Autodesk Inventor part; units mm, degrees
(part 2 of 2)
sketch "스케치20" plane through (0, 6, 0) normal (0, 1, 0) x (1, 0, 0)
  line L0 (-73.8574, -232.5656) -> (-73.8574, -229.8656) projected
  line L1 (-73.8574, -232.5656) -> (-73.8574, -229.8656) projected
  line L2 (-89.8574, -208.2156) -> (-95.8574, -208.2156) projected
  line L3 (-89.8574, -208.2156) -> (-95.8574, -208.2156) projected
  line L4 (-89.8574, -208.2156) -> (-95.8574, -208.2156) projected
  line L5 (-89.8574, -208.2156) -> (-95.8574, -208.2156) projected
  line L6 (-73.8574, -232.5656) -> (-73.8574, -229.8656) projected
  line L7 (-89.8574, -232.5656) -> (-89.8574, -229.8656) projected
  line L8 (-89.8574, -232.5656) -> (-89.8574, -229.8656) projected
  line L9 (-95.8574, -223.2156) -> (-95.8574, -213.2156) projected
  line L10 (-95.8574, -213.2156) -> (-95.8574, -223.2156) projected
  line L11 (-95.8574, -228.2156) -> (-95.8574, -213.2156) projected
  line L12 (-89.8574, -228.2156) -> (-95.8574, -228.2156) projected
  line L13 (-89.8574, -228.2156) -> (-95.8574, -228.2156) projected
  line L14 (-89.8574, -228.2156) -> (-95.8574, -228.2156) projected
  line L15 (-89.8574, -228.2156) -> (-95.8574, -228.2156) projected
  line L16 (-95.8574, -213.2156) -> (-95.8574, -228.2156) projected
  line L17 (-73.8574, -206.5656) -> (-73.8574, -203.8656) projected
  line L18 (-73.8574, -206.5656) -> (-73.8574, -203.8656) projected
  line L19 (-89.8574, -206.5656) -> (-89.8574, -203.8656) projected
  line L20 (-73.8574, -206.5656) -> (-73.8574, -203.8656) projected
  line L21 (-89.8574, -206.5656) -> (-89.8574, -203.8656) projected
  line L22 (43.6426, -213.2156) -> (43.6426, -223.2156) projected
  line L23 (43.6426, -258.2156) -> (43.6426, -223.2156) projected
  line L24 (43.6426, -203.8656) -> (43.6426, -206.5656) projected
  line L25 (27.6426, -203.8656) -> (27.6426, -206.5656) projected
  line L26 (43.6426, -229.8656) -> (43.6426, -232.5656) projected
  line L27 (27.6426, -229.8656) -> (27.6426, -232.5656) projected
  line L28 (43.6426, -203.8656) -> (43.6426, -206.5656) projected
  line L29 (43.6426, -258.2156) -> (43.6426, -223.2156) projected
  line L30 (43.6426, -213.2156) -> (43.6426, -168.8156) projected
  line L31 (43.6426, -175.4656) -> (43.6426, -178.1656) projected
  line L32 (27.6426, -203.8656) -> (27.6426, -206.5656) projected
  line L33 (27.6426, -229.8656) -> (27.6426, -232.5656) projected
  line L34 (27.6426, -203.8656) -> (27.6426, -206.5656) projected
  line L35 (43.6426, -203.8656) -> (43.6426, -206.5656) projected
  line L36 (27.6426, -229.8656) -> (27.6426, -232.5656) projected
  line L37 (43.6426, -229.8656) -> (43.6426, -232.5656) projected
  line L38 (43.6426, -208.2156) -> (49.6426, -208.2156) projected
  line L39 (43.6426, -208.2156) -> (49.6426, -208.2156) projected
  line L40 (49.6426, -223.2156) -> (49.6426, -213.2156) projected
  line L41 (49.6426, -213.2156) -> (49.6426, -223.2156) projected
  line L42 (43.6426, -228.2156) -> (49.6426, -228.2156) projected
  line L43 (43.6426, -228.2156) -> (49.6426, -228.2156) projected
  line L44 (49.6426, -213.2156) -> (49.6426, -223.2156) projected
  line L45 (43.6426, -228.2156) -> (49.6426, -228.2156) projected
  line L46 (43.6426, -228.2156) -> (49.6426, -228.2156) projected
  line L47 (49.6426, -223.2156) -> (49.6426, -213.2156) projected
  line L48 (43.6426, -208.2156) -> (49.6426, -208.2156) projected
  line L49 (43.6426, -208.2156) -> (49.6426, -208.2156) projected
  line L50 (43.6426, -258.2156) -> (43.6426, -223.2156) projected
  line L51 (43.6426, -258.2156) -> (43.6426, -223.2156) projected
  line L52 (43.6426, -229.8656) -> (43.6426, -232.5656) projected
  line L53 (43.6426, -258.2156) -> (43.6426, -223.2156) projected
  line L54 (43.6426, -258.2156) -> (43.6426, -223.2156) projected
  line L55 (1.8926, -153.8156) -> (1.8926, -173.8156) projected
  line L56 (1.8926, -173.8156) -> (-48.1074, -173.8156) projected
  line L57 (-48.1074, -173.8156) -> (-48.1074, -153.8156) projected
  line L58 (-48.1074, -153.8156) -> (1.8926, -153.8156) projected
  line L59 (-67.2574, -135.1156) -> (-67.2574, -137.3156) projected
  line L60 (-67.2574, -137.3156) -> (-72.4574, -137.3156) projected
  line L61 (-72.4574, -137.3156) -> (-72.4574, -135.1156) projected
  line L62 (-72.4574, -135.1156) -> (-67.2574, -135.1156) projected
  line L63 (21.0426, -135.1156) -> (26.2426, -135.1156) projected
  line L64 (26.2426, -135.1156) -> (26.2426, -137.3156) projected
  line L65 (26.2426, -137.3156) -> (21.0426, -137.3156) projected
  line L66 (21.0426, -137.3156) -> (21.0426, -135.1156) projected
  line L67 (-80.7574, -148.2156) -> (-80.7574, -153.4156) projected
  line L68 (-80.7574, -153.4156) -> (-82.9574, -153.4156) projected
  line L69 (-82.9574, -153.4156) -> (-82.9574, -148.2156) projected
  line L70 (-82.9574, -148.2156) -> (-80.7574, -148.2156) projected
  line L71 (34.5426, -148.2156) -> (36.7426, -148.2156) projected
  line L72 (36.7426, -148.2156) -> (36.7426, -153.4156) projected
  line L73 (36.7426, -153.4156) -> (34.5426, -153.4156) projected
  line L74 (34.5426, -153.4156) -> (34.5426, -148.2156) projected
  line L75 (-8.2304, -181.0703) -> (-8.2304, -248.2156) projected
  line L76 (-8.2304, -248.2156) -> (-38.2304, -248.2156) projected
  line L77 (-38.2304, -248.2156) -> (-38.2304, -181.0703) projected
  arc A0 (-36.6425, -180.6156) -> (-38.2304, -181.0703) centre (-36.6425, -183.6156) ccw projected
  line L78 (-36.6425, -180.6156) -> (-9.8183, -180.6156) projected
  arc A1 (-8.2304, -181.0703) -> (-9.8183, -180.6156) centre (-9.8183, -183.6156) ccw projected
  line L79 (43.6426, -258.2156) -> (43.6426, -223.2156) projected
  line L80 (49.6426, -213.2156) -> (49.6426, -223.2156) projected
  line L81 (43.6426, -213.2156) -> (43.6426, -168.8156) projected
  line L82 (49.6426, -158.8156) -> (49.6426, -168.8156) projected
  line L83 (43.6426, -158.8156) -> (43.6426, -128.2156) projected
  line L84 (43.6426, -128.2156) -> (-3.1074, -128.2156) projected
  line L85 (-3.1074, -128.2156) -> (-3.1074, -122.2156) projected
  line L86 (-43.1074, -122.2156) -> (-3.1074, -122.2156) projected
  line L87 (-43.1074, -128.2156) -> (-43.1074, -122.2156) projected
  line L88 (-43.1074, -128.2156) -> (-89.8574, -128.2156) projected
  line L89 (-89.8574, -128.2156) -> (-89.8574, -158.8156) projected
  line L90 (-95.8574, -223.2156) -> (-95.8574, -213.2156) projected
  line L91 (-89.8574, -223.2156) -> (-89.8574, -258.2156) projected
  line L92 (-89.8574, -258.2156) -> (43.6426, -258.2156) projected
  circle A2 centre (-5.9304, -232.7156) radius 1.35 projected
  circle A3 centre (-5.9304, -210.7156) radius 1.35 projected
  circle A4 centre (-5.9304, -188.7156) radius 1.35 projected
  circle A5 centre (-40.5304, -188.7156) radius 1.35 projected
  circle A6 centre (-40.5304, -232.7156) radius 1.35 projected
  circle A7 centre (-40.5304, -210.7156) radius 1.35 projected
  line L93 (1.8926, -173.8156) -> (1.8926, -153.8156) projected
  line L94 (1.8926, -153.8156) -> (-48.1074, -153.8156) projected
  line L95 (-48.1074, -153.8156) -> (-48.1074, -173.8156) projected
  line L96 (-48.1074, -173.8156) -> (1.8926, -173.8156) projected
  line L97 (-67.2574, -137.3156) -> (-67.2574, -135.1156) projected
  line L98 (-67.2574, -135.1156) -> (-72.4574, -135.1156) projected
  line L99 (-72.4574, -135.1156) -> (-72.4574, -137.3156) projected
  line L100 (-72.4574, -137.3156) -> (-67.2574, -137.3156) projected
  line L101 (26.2426, -135.1156) -> (21.0426, -135.1156) projected
  line L102 (21.0426, -135.1156) -> (21.0426, -137.3156) projected
  line L103 (21.0426, -137.3156) -> (26.2426, -137.3156) projected
  line L104 (26.2426, -137.3156) -> (26.2426, -135.1156) projected
  line L105 (-80.7574, -153.4156) -> (-80.7574, -148.2156) projected
  line L106 (-80.7574, -148.2156) -> (-82.9574, -148.2156) projected
  line L107 (-82.9574, -148.2156) -> (-82.9574, -153.4156) projected
  line L108 (-82.9574, -153.4156) -> (-80.7574, -153.4156) projected
  line L109 (36.7426, -148.2156) -> (34.5426, -148.2156) projected
  line L110 (34.5426, -148.2156) -> (34.5426, -153.4156) projected
  line L111 (34.5426, -153.4156) -> (36.7426, -153.4156) projected
  line L112 (36.7426, -153.4156) -> (36.7426, -148.2156) projected
  line L113 (-8.2304, -181.0703) -> (-8.2304, -248.2156) projected
  arc A8 (-8.2304, -181.0703) -> (-9.8183, -180.6156) centre (-9.8183, -183.6156) ccw projected
  line L114 (-36.6425, -180.6156) -> (-9.8183, -180.6156) projected
  arc A9 (-36.6425, -180.6156) -> (-38.2304, -181.0703) centre (-36.6425, -183.6156) ccw projected
  line L115 (-38.2304, -248.2156) -> (-38.2304, -181.0703) projected
  line L116 (-8.2304, -248.2156) -> (-38.2304, -248.2156) projected
  line L117 (43.6426, -158.8156) -> (43.6426, -128.2156) projected
  line L118 (-89.8574, -258.2156) -> (43.6426, -258.2156) projected
  line L119 (-89.8574, -128.2156) -> (-89.8574, -158.8156) projected
  line L120 (-95.8574, -213.2156) -> (-95.8574, -223.2156) projected
  line L121 (-89.8574, -168.8156) -> (-89.8574, -213.2156) projected
  line L122 (-43.1074, -128.2156) -> (-89.8574, -128.2156) projected
  line L123 (-43.1074, -128.2156) -> (-43.1074, -122.2156) projected
  line L124 (-3.1074, -122.2156) -> (-43.1074, -122.2156) projected
  line L125 (-3.1074, -128.2156) -> (-3.1074, -122.2156) projected
  line L126 (43.6426, -128.2156) -> (-3.1074, -128.2156) projected
  line L127 (43.6426, -258.2156) -> (43.6426, -223.2156) projected
  line L128 (49.6426, -168.8156) -> (49.6426, -158.8156) projected
  line L129 (43.6426, -213.2156) -> (43.6426, -168.8156) projected
  line L130 (49.6426, -223.2156) -> (49.6426, -213.2156) projected
  circle A10 centre (-5.9304, -232.7156) radius 1.35 projected
  circle A11 centre (-5.9304, -210.7156) radius 1.35 projected
  circle A12 centre (-5.9304, -188.7156) radius 1.35 projected
  circle A13 centre (-40.5304, -188.7156) radius 1.35 projected
  circle A14 centre (-40.5304, -232.7156) radius 1.35 projected
  circle A15 centre (-40.5304, -210.7156) radius 1.35 projected
  line L131 (-89.8574, -203.8656) -> (-73.8574, -203.8656) projected
  line L132 (-89.8574, -206.5656) -> (-73.8574, -206.5656) projected
  line L133 (-89.8574, -229.8656) -> (-73.8574, -229.8656) projected
  line L134 (-89.8574, -232.5656) -> (-73.8574, -232.5656) projected
  line L135 (43.6426, -203.8656) -> (27.6426, -203.8656) projected
  line L136 (43.6426, -206.5656) -> (27.6426, -206.5656) projected
  line L137 (43.6426, -229.8656) -> (27.6426, -229.8656) projected
  line L138 (43.6426, -232.5656) -> (27.6426, -232.5656) projected
  line L139 (-82.9574, -207.8156) -> (-80.7574, -207.8156)
  line L140 (-80.7574, -207.8156) -> (-80.7574, -202.6156)
  line L141 (-80.7574, -202.6156) -> (-82.9574, -202.6156)
  line L142 (-82.9574, -202.6156) -> (-82.9574, -207.8156)
  line L143 (-82.9574, -207.8156) -> (-80.7574, -202.6156) construction
  line L144 (-80.7574, -207.8156) -> (-82.9574, -202.6156) construction
  line L145 (-82.9574, -233.9656) -> (-80.7574, -233.9656)
  line L146 (-80.7574, -233.9656) -> (-80.7574, -228.7656)
  line L147 (-80.7574, -228.7656) -> (-82.9574, -228.7656)
  line L148 (-82.9574, -228.7656) -> (-82.9574, -233.9656)
  line L149 (-82.9574, -233.9656) -> (-80.7574, -228.7656) construction
  line L150 (-80.7574, -233.9656) -> (-82.9574, -228.7656) construction
  line L151 (34.5426, -207.8156) -> (36.7426, -207.8156)
  line L152 (36.7426, -207.8156) -> (36.7426, -202.6156)
  line L153 (36.7426, -202.6156) -> (34.5426, -202.6156)
  line L154 (34.5426, -202.6156) -> (34.5426, -207.8156)
  line L155 (34.5426, -207.8156) -> (36.7426, -202.6156) construction
  line L156 (36.7426, -207.8156) -> (34.5426, -202.6156) construction
  line L157 (34.5426, -233.9656) -> (36.7426, -233.9656)
  line L158 (36.7426, -233.9656) -> (36.7426, -228.7656)
  line L159 (36.7426, -228.7656) -> (34.5426, -228.7656)
  line L160 (34.5426, -228.7656) -> (34.5426, -233.9656)
  line L161 (34.5426, -233.9656) -> (36.7426, -228.7656) construction
  line L162 (36.7426, -233.9656) -> (34.5426, -228.7656) construction
  line L163 (43.6426, -213.2156) -> (49.6426, -213.2156) projected
  line L164 (43.6426, -223.2156) -> (49.6426, -223.2156) projected
  line L165 (43.6426, -223.2156) -> (49.6426, -223.2156) projected
  line L166 (43.6426, -213.2156) -> (49.6426, -213.2156) projected
  line L167 (43.6426, -158.8156) -> (43.6426, -128.2156) projected
  line L168 (43.6426, -158.8156) -> (43.6426, -128.2156) projected
  line L169 (43.6426, -213.2156) -> (43.6426, -168.8156) projected
  line L170 (43.6426, -213.2156) -> (43.6426, -168.8156) projected
  line L171 (43.6426, -158.8156) -> (43.6426, -128.2156) projected
  line L172 (43.6426, -158.8156) -> (43.6426, -128.2156) projected
  line L173 (43.6426, -213.2156) -> (43.6426, -168.8156) projected
  line L174 (43.6426, -258.2156) -> (43.6426, -223.2156) projected
  line L175 (43.6426, -158.8156) -> (49.6426, -158.8156) projected
  line L176 (43.6426, -168.8156) -> (49.6426, -168.8156) projected
  line L177 (43.6426, -168.8156) -> (49.6426, -168.8156) projected
  line L178 (43.6426, -158.8156) -> (49.6426, -158.8156) projected
  line L179 (-89.8574, -223.2156) -> (-89.8574, -258.2156) projected
  line L180 (-89.8574, -168.8156) -> (-95.8574, -168.8156) projected
  line L181 (-95.8574, -158.8156) -> (-95.8574, -168.8156) projected
  line L182 (-89.8574, -158.8156) -> (-95.8574, -158.8156) projected
  line L183 (-89.8574, -158.8156) -> (-95.8574, -158.8156) projected
  line L184 (-95.8574, -168.8156) -> (-95.8574, -158.8156) projected
  line L185 (-89.8574, -168.8156) -> (-95.8574, -168.8156) projected
  line L186 (-89.8574, -168.8156) -> (-89.8574, -213.2156) projected
  line L187 (-89.8574, -223.2156) -> (-95.8574, -223.2156) projected
  line L188 (-89.8574, -213.2156) -> (-95.8574, -213.2156) projected
  line L189 (-89.8574, -213.2156) -> (-95.8574, -213.2156) projected
  line L190 (-89.8574, -223.2156) -> (-95.8574, -223.2156) projected
  point P0 (0, 0)
  point P1 (43.6426, -173.8156)
  point P2 (-81.8574, -205.2156)
  point P3 (-81.8574, -231.3656)
  point P4 (35.6426, -205.2156)
  point P5 (35.6426, -231.3656)
  dimension "d155" = 2.2
  dimension "d156" = 5.2
  dimension "d157" = 2.2
  dimension "d158" = 5.2
  dimension "d159" = 2.2
  dimension "d160" = 5.2
  dimension "d161" = 2.2
  dimension "d162" = 5.2
  constraints: 48 end point, 8 midpoint, 8 parallel, 4 horizontal, 4 perpendicular, 7 other
  measures "d155" distance of L141.end L140.end
  measures "d156" distance of L140.end L139.end
  measures "d157" distance of L147.end L146.end
  measures "d158" distance of L146.end L145.end
  measures "d159" distance of L153.end L152.end
  measures "d160" distance of L152.end L151.end
  measures "d161" distance of L159.end L158.end
  measures "d162" distance of L158.end L157.end
extrude "돌출18" cut sketch "스케치20" against normal blind 16 contours L146 L145 L148 L134 | L134 L148 L133 L146 | L133 L148 L147 L146 | L158 L157 L160 L138 | L138 L160 L137 L158 | L137 L160 L159 L158 | L142 L131 L140 L132 | L132 L140 L139 L142 | L142 L141 L140 L131 | L152 L151 L154 L136 | L136 L154 L135 L152 | L135 L154 L153 L152
sketch "스케치22" plane through (0, 6, 0) normal (0, 1, 0) x (1, 0, 0)
  line L0 (36.7426, -207.8156) -> (34.5426, -207.8156) projected
  line L1 (34.5426, -207.8156) -> (34.5426, -202.6156) projected
  line L2 (34.5426, -202.6156) -> (36.7426, -202.6156) projected
  line L3 (36.7426, -202.6156) -> (36.7426, -207.8156) projected
  line L4 (-80.7574, -233.9656) -> (-82.9574, -233.9656) projected
  line L5 (-82.9574, -233.9656) -> (-82.9574, -228.7656) projected
  line L6 (-82.9574, -228.7656) -> (-80.7574, -228.7656) projected
  line L7 (-80.7574, -228.7656) -> (-80.7574, -233.9656) projected
  line L8 (36.7426, -233.9656) -> (34.5426, -233.9656) projected
  line L9 (34.5426, -233.9656) -> (34.5426, -228.7656) projected
  line L10 (34.5426, -228.7656) -> (36.7426, -228.7656) projected
  line L11 (36.7426, -228.7656) -> (36.7426, -233.9656) projected
  line L12 (-80.7574, -207.8156) -> (-82.9574, -207.8156) projected
  line L13 (-82.9574, -207.8156) -> (-82.9574, -202.6156) projected
  line L14 (-82.9574, -202.6156) -> (-80.7574, -202.6156) projected
  line L15 (-80.7574, -202.6156) -> (-80.7574, -207.8156) projected
  line L16 (1.8926, -153.8156) -> (1.8926, -173.8156) projected
  line L17 (1.8926, -173.8156) -> (-48.1074, -173.8156) projected
  line L18 (-48.1074, -173.8156) -> (-48.1074, -153.8156) projected
  line L19 (-48.1074, -153.8156) -> (1.8926, -153.8156) projected
  line L20 (34.5426, -148.2156) -> (36.7426, -148.2156) projected
  line L21 (36.7426, -148.2156) -> (36.7426, -153.4156) projected
  line L22 (36.7426, -153.4156) -> (34.5426, -153.4156) projected
  line L23 (34.5426, -153.4156) -> (34.5426, -148.2156) projected
  line L24 (-80.7574, -148.2156) -> (-80.7574, -153.4156) projected
  line L25 (-80.7574, -153.4156) -> (-82.9574, -153.4156) projected
  line L26 (-82.9574, -153.4156) -> (-82.9574, -148.2156) projected
  line L27 (-82.9574, -148.2156) -> (-80.7574, -148.2156) projected
  line L28 (36.7426, -179.4156) -> (34.5426, -179.4156) projected
  line L29 (34.5426, -179.4156) -> (34.5426, -174.2156) projected
  line L30 (34.5426, -174.2156) -> (36.7426, -174.2156) projected
  line L31 (36.7426, -174.2156) -> (36.7426, -179.4156) projected
  line L32 (21.0426, -135.1156) -> (26.2426, -135.1156) projected
  line L33 (26.2426, -135.1156) -> (26.2426, -137.3156) projected
  line L34 (26.2426, -137.3156) -> (21.0426, -137.3156) projected
  line L35 (21.0426, -137.3156) -> (21.0426, -135.1156) projected
  line L36 (-67.2574, -135.1156) -> (-67.2574, -137.3156) projected
  line L37 (-67.2574, -137.3156) -> (-72.4574, -137.3156) projected
  line L38 (-72.4574, -137.3156) -> (-72.4574, -135.1156) projected
  line L39 (-72.4574, -135.1156) -> (-67.2574, -135.1156) projected
  line L40 (-80.7574, -179.4156) -> (-82.9574, -179.4156) projected
  line L41 (-82.9574, -179.4156) -> (-82.9574, -174.2156) projected
  line L42 (-82.9574, -174.2156) -> (-80.7574, -174.2156) projected
  line L43 (-80.7574, -174.2156) -> (-80.7574, -179.4156) projected
  line L44 (-8.2304, -181.0703) -> (-8.2304, -248.2156) projected
  line L45 (-8.2304, -248.2156) -> (-38.2304, -248.2156) projected
  line L46 (-38.2304, -248.2156) -> (-38.2304, -181.0703) projected
  arc A0 (-36.6425, -180.6156) -> (-38.2304, -181.0703) centre (-36.6425, -183.6156) ccw projected
  line L47 (-36.6425, -180.6156) -> (-9.8183, -180.6156) projected
  arc A1 (-8.2304, -181.0703) -> (-9.8183, -180.6156) centre (-9.8183, -183.6156) ccw projected
  line L48 (43.6426, -258.2156) -> (43.6426, -223.2156) projected
  line L49 (49.6426, -213.2156) -> (49.6426, -223.2156) projected
  line L50 (43.6426, -213.2156) -> (43.6426, -168.8156) projected
  line L51 (49.6426, -158.8156) -> (49.6426, -168.8156) projected
  line L52 (43.6426, -158.8156) -> (43.6426, -128.2156) projected
  line L53 (43.6426, -128.2156) -> (-3.1074, -128.2156) projected
  line L54 (-3.1074, -128.2156) -> (-3.1074, -122.2156) projected
  line L55 (-43.1074, -122.2156) -> (-3.1074, -122.2156) projected
  line L56 (-43.1074, -128.2156) -> (-43.1074, -122.2156) projected
  line L57 (-43.1074, -128.2156) -> (-89.8574, -128.2156) projected
  line L58 (-89.8574, -128.2156) -> (-89.8574, -158.8156) projected
  line L59 (-95.8574, -223.2156) -> (-95.8574, -213.2156) projected
  line L60 (-89.8574, -223.2156) -> (-89.8574, -258.2156) projected
  line L61 (-89.8574, -258.2156) -> (43.6426, -258.2156) projected
  circle A2 centre (-5.9304, -232.7156) radius 1.35 projected
  circle A3 centre (-5.9304, -210.7156) radius 1.35 projected
  circle A4 centre (-5.9304, -188.7156) radius 1.35 projected
  circle A5 centre (-40.5304, -188.7156) radius 1.35 projected
  circle A6 centre (-40.5304, -232.7156) radius 1.35 projected
  circle A7 centre (-40.5304, -210.7156) radius 1.35 projected
  line L62 (1.8926, -188.7156) -> (21.8926, -188.7156)
  line L63 (21.8926, -188.7156) -> (21.8926, -201.7156)
  line L64 (21.8926, -201.7156) -> (1.8926, -201.7156)
  line L65 (1.8926, -201.7156) -> (1.8926, -188.7156)
  line L66 (-48.1074, -188.7156) -> (-68.1074, -188.7156)
  line L67 (-68.1074, -188.7156) -> (-68.1074, -201.7156)
  line L68 (-68.1074, -201.7156) -> (-48.1074, -201.7156)
  line L69 (-48.1074, -201.7156) -> (-48.1074, -188.7156)
  line L70 (21.8926, -188.7156) -> (36.8926, -188.7156)
  line L71 (36.8926, -188.7156) -> (36.8926, -196.7156)
  line L72 (36.8926, -196.7156) -> (21.8926, -196.7156)
  line L73 (21.8926, -196.7156) -> (21.8926, -188.7156)
  line L74 (-68.1074, -188.7156) -> (-83.1074, -188.7156)
  line L75 (-83.1074, -188.7156) -> (-83.1074, -196.7156)
  line L76 (-83.1074, -196.7156) -> (-68.1074, -196.7156)
  line L77 (-68.1074, -196.7156) -> (-68.1074, -188.7156)
  line L78 (43.6426, -223.2156) -> (49.6426, -223.2156) projected
  line L79 (43.6426, -213.2156) -> (49.6426, -213.2156) projected
  line L80 (43.6426, -168.8156) -> (49.6426, -168.8156) projected
  line L81 (43.6426, -158.8156) -> (49.6426, -158.8156) projected
  line L82 (-89.8574, -158.8156) -> (-95.8574, -158.8156) projected
  line L83 (-95.8574, -168.8156) -> (-95.8574, -158.8156) projected
  line L84 (-89.8574, -168.8156) -> (-95.8574, -168.8156) projected
  line L85 (-89.8574, -168.8156) -> (-89.8574, -213.2156) projected
  line L86 (-89.8574, -213.2156) -> (-95.8574, -213.2156) projected
  line L87 (-89.8574, -223.2156) -> (-95.8574, -223.2156) projected
  point P0 (0, 0)
  dimension "d168" = 20
  dimension "d169" = 13
  dimension "d170" = 20
  dimension "d171" = 15
  dimension "d172" = 8
  dimension "d173" = 15
  dimension "d174" = 8
  constraints: 32 end point, 8 parallel, 4 horizontal, 4 perpendicular, 2 point on line
  measures "d168" distance of L63.end L64.end
  measures "d169" distance of L62.end L63.end
  measures "d170" distance of L68.end L67.end
  measures "d171" distance of L71.end L72.end
  measures "d172" distance of L70.end L71.end
  measures "d173" distance of L76.end L75.end
  measures "d174" distance of L75.end L74.end
extrude "돌출19" cut sketch "스케치22" against normal blind 10 contours L70 L71 L72 L63 | L67 L76 L75 L74
sketch "스케치23" plane through (0, 6, 0) normal (0, 1, 0) x (1, 0, 0)
  line L0 (21.8926, -196.7156) -> (21.8926, -188.7156) projected
  line L1 (21.8926, -188.7156) -> (36.8926, -188.7156) projected
  line L2 (36.8926, -188.7156) -> (36.8926, -196.7156) projected
  line L3 (36.8926, -196.7156) -> (21.8926, -196.7156) projected
  line L4 (-68.1074, -188.7156) -> (-68.1074, -196.7156) projected
  line L5 (-68.1074, -196.7156) -> (-83.1074, -196.7156) projected
  line L6 (-83.1074, -196.7156) -> (-83.1074, -188.7156) projected
  line L7 (-83.1074, -188.7156) -> (-68.1074, -188.7156) projected
  line L8 (36.7426, -207.8156) -> (34.5426, -207.8156) projected
  line L9 (34.5426, -207.8156) -> (34.5426, -202.6156) projected
  line L10 (34.5426, -202.6156) -> (36.7426, -202.6156) projected
  line L11 (36.7426, -202.6156) -> (36.7426, -207.8156) projected
  line L12 (-80.7574, -233.9656) -> (-82.9574, -233.9656) projected
  line L13 (-82.9574, -233.9656) -> (-82.9574, -228.7656) projected
  line L14 (-82.9574, -228.7656) -> (-80.7574, -228.7656) projected
  line L15 (-80.7574, -228.7656) -> (-80.7574, -233.9656) projected
  line L16 (36.7426, -233.9656) -> (34.5426, -233.9656) projected
  line L17 (34.5426, -233.9656) -> (34.5426, -228.7656) projected
  line L18 (34.5426, -228.7656) -> (36.7426, -228.7656) projected
  line L19 (36.7426, -228.7656) -> (36.7426, -233.9656) projected
  line L20 (-80.7574, -207.8156) -> (-82.9574, -207.8156) projected
  line L21 (-82.9574, -207.8156) -> (-82.9574, -202.6156) projected
  line L22 (-82.9574, -202.6156) -> (-80.7574, -202.6156) projected
  line L23 (-80.7574, -202.6156) -> (-80.7574, -207.8156) projected
  line L24 (1.8926, -153.8156) -> (1.8926, -173.8156) projected
  line L25 (1.8926, -173.8156) -> (-48.1074, -173.8156) projected
  line L26 (-48.1074, -173.8156) -> (-48.1074, -153.8156) projected
  line L27 (-48.1074, -153.8156) -> (1.8926, -153.8156) projected
  line L28 (34.5426, -148.2156) -> (36.7426, -148.2156) projected
  line L29 (36.7426, -148.2156) -> (36.7426, -153.4156) projected
  line L30 (36.7426, -153.4156) -> (34.5426, -153.4156) projected
  line L31 (34.5426, -153.4156) -> (34.5426, -148.2156) projected
  line L32 (-80.7574, -148.2156) -> (-80.7574, -153.4156) projected
  line L33 (-80.7574, -153.4156) -> (-82.9574, -153.4156) projected
  line L34 (-82.9574, -153.4156) -> (-82.9574, -148.2156) projected
  line L35 (-82.9574, -148.2156) -> (-80.7574, -148.2156) projected
  line L36 (36.7426, -179.4156) -> (34.5426, -179.4156) projected
  line L37 (34.5426, -179.4156) -> (34.5426, -174.2156) projected
  line L38 (34.5426, -174.2156) -> (36.7426, -174.2156) projected
  line L39 (36.7426, -174.2156) -> (36.7426, -179.4156) projected
  line L40 (21.0426, -135.1156) -> (26.2426, -135.1156) projected
  line L41 (26.2426, -135.1156) -> (26.2426, -137.3156) projected
  line L42 (26.2426, -137.3156) -> (21.0426, -137.3156) projected
  line L43 (21.0426, -137.3156) -> (21.0426, -135.1156) projected
  line L44 (-67.2574, -135.1156) -> (-67.2574, -137.3156) projected
  line L45 (-67.2574, -137.3156) -> (-72.4574, -137.3156) projected
  line L46 (-72.4574, -137.3156) -> (-72.4574, -135.1156) projected
  line L47 (-72.4574, -135.1156) -> (-67.2574, -135.1156) projected
  line L48 (-80.7574, -179.4156) -> (-82.9574, -179.4156) projected
  line L49 (-82.9574, -179.4156) -> (-82.9574, -174.2156) projected
  line L50 (-82.9574, -174.2156) -> (-80.7574, -174.2156) projected
  line L51 (-80.7574, -174.2156) -> (-80.7574, -179.4156) projected
  line L52 (-8.2304, -181.0703) -> (-8.2304, -248.2156) projected
  line L53 (-8.2304, -248.2156) -> (-38.2304, -248.2156) projected
  line L54 (-38.2304, -248.2156) -> (-38.2304, -181.0703) projected
  arc A0 (-36.6425, -180.6156) -> (-38.2304, -181.0703) centre (-36.6425, -183.6156) ccw projected
  line L55 (-36.6425, -180.6156) -> (-9.8183, -180.6156) projected
  arc A1 (-8.2304, -181.0703) -> (-9.8183, -180.6156) centre (-9.8183, -183.6156) ccw projected
  line L56 (43.6426, -258.2156) -> (43.6426, -223.2156) projected
  line L57 (43.6426, -223.2156) -> (49.6426, -223.2156) projected
  line L58 (49.6426, -213.2156) -> (49.6426, -223.2156) projected
  line L59 (43.6426, -213.2156) -> (49.6426, -213.2156) projected
  line L60 (43.6426, -213.2156) -> (43.6426, -168.8156) projected
  line L61 (43.6426, -168.8156) -> (49.6426, -168.8156) projected
  line L62 (49.6426, -158.8156) -> (49.6426, -168.8156) projected
  line L63 (43.6426, -158.8156) -> (49.6426, -158.8156) projected
  line L64 (43.6426, -158.8156) -> (43.6426, -128.2156) projected
  line L65 (43.6426, -128.2156) -> (-3.1074, -128.2156) projected
  line L66 (-3.1074, -128.2156) -> (-3.1074, -122.2156) projected
  line L67 (-43.1074, -122.2156) -> (-3.1074, -122.2156) projected
  line L68 (-43.1074, -128.2156) -> (-43.1074, -122.2156) projected
  line L69 (-43.1074, -128.2156) -> (-89.8574, -128.2156) projected
  line L70 (-89.8574, -128.2156) -> (-89.8574, -158.8156) projected
  line L71 (-89.8574, -158.8156) -> (-95.8574, -158.8156) projected
  line L72 (-95.8574, -168.8156) -> (-95.8574, -158.8156) projected
  line L73 (-89.8574, -168.8156) -> (-95.8574, -168.8156) projected
  line L74 (-89.8574, -168.8156) -> (-89.8574, -213.2156) projected
  line L75 (-89.8574, -213.2156) -> (-95.8574, -213.2156) projected
  line L76 (-95.8574, -223.2156) -> (-95.8574, -213.2156) projected
  line L77 (-89.8574, -223.2156) -> (-95.8574, -223.2156) projected
  line L78 (-89.8574, -223.2156) -> (-89.8574, -258.2156) projected
  line L79 (-89.8574, -258.2156) -> (43.6426, -258.2156) projected
  circle A2 centre (-5.9304, -232.7156) radius 1.35 projected
  circle A3 centre (-5.9304, -210.7156) radius 1.35 projected
  circle A4 centre (-5.9304, -188.7156) radius 1.35 projected
  circle A5 centre (-40.5304, -188.7156) radius 1.35 projected
  circle A6 centre (-40.5304, -232.7156) radius 1.35 projected
  circle A7 centre (-40.5304, -210.7156) radius 1.35 projected
  line L80 (-89.8574, -228.2156) -> (-95.8574, -228.2156)
  line L81 (-95.8574, -228.2156) -> (-95.8574, -208.2156)
  line L82 (-95.8574, -208.2156) -> (-89.8574, -208.2156)
  line L83 (-89.8574, -208.2156) -> (-89.8574, -228.2156)
  line L84 (-89.8574, -228.2156) -> (-95.8574, -208.2156) construction
  line L85 (-95.8574, -228.2156) -> (-89.8574, -208.2156) construction
  line L86 (-89.8574, -173.8156) -> (-95.8574, -173.8156)
  line L87 (-95.8574, -173.8156) -> (-95.8574, -153.8156)
  line L88 (-95.8574, -153.8156) -> (-89.8574, -153.8156)
  line L89 (-89.8574, -153.8156) -> (-89.8574, -173.8156)
  line L90 (-89.8574, -173.8156) -> (-95.8574, -153.8156) construction
  line L91 (-95.8574, -173.8156) -> (-89.8574, -153.8156) construction
  line L92 (49.6426, -228.2156) -> (43.6426, -228.2156)
  line L93 (43.6426, -228.2156) -> (43.6426, -208.2156)
  line L94 (43.6426, -208.2156) -> (49.6426, -208.2156)
  line L95 (49.6426, -208.2156) -> (49.6426, -228.2156)
  line L96 (49.6426, -228.2156) -> (43.6426, -208.2156) construction
  line L97 (43.6426, -228.2156) -> (49.6426, -208.2156) construction
  line L98 (49.6426, -173.8156) -> (43.6426, -173.8156)
  line L99 (43.6426, -173.8156) -> (43.6426, -153.8156)
  line L100 (43.6426, -153.8156) -> (49.6426, -153.8156)
  line L101 (49.6426, -153.8156) -> (49.6426, -173.8156)
  line L102 (49.6426, -173.8156) -> (43.6426, -153.8156) construction
  line L103 (43.6426, -173.8156) -> (49.6426, -153.8156) construction
  point P0 (0, 0)
  point P1 (-92.8574, -218.2156)
  point P2 (-92.8574, -163.8156)
  point P3 (46.6426, -218.2156)
  point P4 (46.6426, -163.8156)
  dimension "d183" = 20
  dimension "d184" = 20
  constraints: 48 end point, 8 midpoint, 8 parallel, 5 point on line, 4 horizontal, 4 perpendicular
  measures "d183" distance of L80.end L81.end
  measures "d184" distance of L86.end L87.end
extrude "돌출20" add sketch "스케치23" against normal blind 6 contours L56 L57 L95 L92 | L93 L59 L58 L57 | L80 L81 L77 L78 | L60 L94 L95 L59 | L77 L76 L75 L83 | L75 L81 L82 L74 | L60 L61 L101 L98 | L99 L63 L62 L61 | L86 L87 L73 L74 | L64 L100 L101 L63 | L73 L72 L71 L89 | L71 L87 L88 L70
